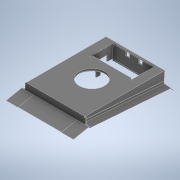
# Autodesk Inventor part: horni-cast
Saved by Autodesk Inventor 2022 (Build 260153000, 153)
## iProperties
Created: 2022-11-28
Part Number: horni-cast
Material: Generic
Document SubType Name: Modeling
Designer: matys
Density: 1 g/cm^3
Appearance: Gray
Author: matys
Autodesk Inventor part; units mm, degrees
ref_plane "YZ Plane" through (0, 0, 0) normal (1, 0, 0) x (0, 1, 0)
ref_plane "XZ Plane" through (0, 0, 0) normal (0, 1, 0) x (-1, 0, 0)
ref_plane "XY Plane" through (0, 0, 0) normal (0, 0, 1) x (1, 0, 0)
sketch "Sketch1" plane through (0, 0, 0) normal (0, 1, 0) x (-1, 0, 0)
  line L0 (0, 0) -> (0, -212.0143)
  line L1 (0, -212.0143) -> (140, -212.0143)
  line L2 (140, -212.0143) -> (140, 0)
  line L3 (140, 0) -> (0, 0)
  dimension "d0" = 212.0143
  dimension "d1" = 140
  constraints: 8 end point, 3 perpendicular, 1 vertical
  measures "d0" distance of L0.start L0.end
  measures "d1" distance of L0.end L1.end
extrude "Extrusion1" add sketch "Sketch1" along normal blind 2.5
sketch "Sketch2" plane through (0, 0, 0) normal (0, -1, 0) x (1, 0, 0)
  line L0 (0, 0) -> (0, -212.0143) projected
  line L1 (0, -212.0143) -> (0, -208.8143)
  line L2 (0, -212.0143) -> (-140, -212.0143) projected
  line L3 (-140, -208.8143) -> (-140, -212.0143)
  line L4 (-140, -212.0143) -> (0, -212.0143)
  line L5 (0, -212.0143) -> (0, -205.5643)
  line L6 (0, -205.5643) -> (-140, -205.5643)
  line L7 (-140, -205.5643) -> (-140, -212.0143)
  dimension "d5" = 6.45
  constraints: 12 end point, 3 perpendicular, 2 point on line
  measures "d5" distance of L0.end L5.end
extrude "Extrusion2" add sketch "Sketch2" along normal blind 40.4609
sketch "Sketch3" plane through (0, 2.5, 0) normal (1, 0, 0) x (0, 0, -1)
  line L0 (0, 0) -> (212.0143, 0) projected
  line L1 (212.0143, 0) -> (208.8143, 0)
  line L2 (212.0143, -42.9609) -> (205.5643, -42.9609) projected
  line L3 (208.8143, 0) -> (208.8143, -2.5)
  line L4 (205.5643, -2.5) -> (0, -2.5) projected
  line L5 (208.8143, -2.5) -> (205.5643, -2.5)
  line L6 (212.0143, 0) -> (209.3663, -37.8675)
  line L7 (212.0143, 0) -> (212.0143, -42.9609) projected
  line L8 (212.0143, 0) -> (209.3663, -37.8675)
  line L9 (209.3663, -37.8675) -> (205.5643, -37.8675)
  line L10 (205.5643, -2.5) -> (205.5643, -42.9609) projected
  line L11 (209.3663, -37.8675) -> (207.8663, -37.8675)
  line L12 (209.3663, -37.8675) -> (212.0143, -37.8675)
  line L13 (207.8663, -37.8675) -> (207.304, -40.3035)
  line L14 (207.304, -40.3035) -> (205.5643, -40.2123)
  line L15 (206.3702, -37.7629) -> (205.8078, -40.1988)
  line L16 (206.3702, -37.7629) -> (208.8143, -2.5)
  line L17 (212.0143, -42.9609) -> (205.5643, -42.9609)
  line L18 (205.5643, -42.9609) -> (205.5643, -2.5)
  line L19 (205.5643, -2.5) -> (212.0143, -2.5)
  line L20 (212.0143, -2.5) -> (212.0143, -42.9609)
  line L21 (212.0143, -2.5) -> (208.8143, -2.5)
  line L22 (208.8143, -2.5) -> (208.8143, 0)
  line L23 (208.8143, 0) -> (212.0143, 0)
  line L24 (212.0143, 0) -> (212.0143, -2.5)
  line L25 (205.8078, -40.1988) -> (205.7916, -40.2692)
  point P0 (206.3461, -37.8675)
  point P1 (205.8019, -40.2247)
  dimension "d8" = 3.2
  dimension "d9" = 86
  dimension "d10" = 37.8675
  dimension "d11" = 37.96
  dimension "d12" = 1.5
  dimension "d14" = 2.5
  dimension "d15" = 100
  dimension "d17" = 2.5
  constraints: 42 end point, 6 point on line, 4 parallel, 3 horizontal, 3 perpendicular, 1 vertical
  measures "d8" distance of L0.end L1.end
  measures "d9" angle of L0 L6
  measures "d10" vertical distance of L6.end L0.end
  measures "d11" distance of L6.end L0.end
  measures "d12" distance of L11.start L11.end
  measures "d14" distance of L13.start L13.end
  measures "d15" angle of L13 L14
  measures "d17" distance of L15.start L15.end
extrude "Extrusion3" cut sketch "Sketch3" against normal through all contours L7 L19 L6 | L16 L15 L9 L10 L5 | L19 L7 L12 L6 | L12 L7 L2 L10 L14 L13 L9 | L9 L15 L25 L14 L10
sketch "Sketch4" plane through (0, 2.5, -212.0143) normal (0, -0.0697565, -0.9975641) x (-1, 0, 0)
  line L0 (0, 0) -> (140, 0) projected
  line L1 (0, 0) -> (140, 0)
  line L2 (140, 0) -> (70, 0)
  line L3 (70, 0) -> (70, -46.5203)
  line L4 (70, 0) -> (120, 0)
  line L5 (120, 0) -> (120, -40.5339)
  line L6 (0, -40.5339) -> (140, -40.5339) projected
  line L7 (120, -40.5339) -> (20, -40.5339)
  line L8 (20, -40.5339) -> (20, 0)
  line L9 (0, -38.0646) -> (140, -38.0646) projected
  line L10 (20, -38.0646) -> (20, -33.0646)
  line L11 (0, -37.96) -> (0, 0) projected
  line L12 (0, -2.7171) -> (0, -38.0646) projected
  line L13 (0, -38.0646) -> (0, -30.0646)
  line L14 (0, -30.0646) -> (20, -30.0646)
  line L15 (0, -30.0646) -> (0, -29.0646)
  line L16 (0, -29.0646) -> (20, -29.0646)
  line L17 (0, -29.0646) -> (0, -46.3446)
  line L18 (0, -46.3446) -> (20, -46.3446)
  line L19 (20, -46.3446) -> (20, -40.5339)
  line L20 (0, -38.0646) -> (0, -40.5601) projected
  line L21 (0, -38.0646) -> (20, -37.96)
  point P0 (0, -17.2833)
  point P1 (0, -29.0646)
  point P2 (0, -38.0646)
  point P3 (0, -40.5339)
  point P4 (20, -40.5339)
  point P5 (0, -38.0646)
  dimension "d20" = 50
  dimension "d21" = 100
  dimension "d23" = 8
  dimension "d24" = 1
  dimension "d25" = 17.28
  constraints: 32 end point, 11 point on line, 6 perpendicular, 2 vertical, 1 collinear, 1 horizontal, 1 midpoint
  measures "d20" distance of L2.end L4.end
  measures "d21" distance of L5.end L7.end
  measures "d23" distance of L9.start L13.end
  measures "d24" distance of L13.end L15.end
  measures "d25" distance of L15.end L17.end
extrude "Extrusion4" add sketch "Sketch4" along normal blind 16 contours L8 L14 L11 L16 | L8 L21 L12 L11 L14 | L9 L21 L8 | L8 L6 L17 L9 | L19 L18 L17 L6
sketch "Sketch5" plane through (0, 2.5, 0) normal (1, 0, 0) x (0, 0, -1)
  line L0 (207.304, -40.3035) -> (207.8663, -37.8675) projected
  line L1 (207.8663, -37.8675) -> (209.3663, -37.8675) projected
  line L2 (207.8663, -37.8675) -> (209.3663, -37.8675)
  line L3 (209.9869, -28.9938) -> (225.9479, -30.1099) projected
  line L4 (209.3663, -37.8675) -> (209.9869, -28.9938)
  line L5 (209.9869, -28.9938) -> (209.9171, -29.9914)
  line L6 (212.0143, 0) -> (209.3663, -37.8675) projected
  line L7 (225.9479, -30.1099) -> (224.7425, -47.3478) projected
  line L8 (224.7425, -47.3478) -> (224.8122, -46.3503)
  line L9 (224.8122, -46.3503) -> (209.9869, -28.9938)
  line L10 (209.9869, -28.9938) -> (209.9171, -29.9914)
  line L11 (209.9171, -29.9914) -> (224.7425, -47.3478)
  line L12 (209.9869, -28.9938) -> (209.7776, -31.9865)
  line L13 (209.9869, -28.9938) -> (209.3663, -37.8675) projected
  line L14 (209.7776, -31.9865) -> (211.7384, -32.1236)
  line L15 (211.7384, -32.1236) -> (209.3663, -37.8675)
  line L16 (225.9479, -30.1099) -> (209.9869, -28.9938)
  line L17 (225.9479, -30.1099) -> (224.8122, -46.3503)
  line L18 (209.3663, -37.8675) -> (208.7815, -46.2317) projected
  line L19 (224.7425, -47.3478) -> (208.7815, -46.2317)
  line L20 (208.7815, -46.2317) -> (209.3663, -37.8675)
  point P0 (0, -2.5)
  dimension "d28" = 1
  dimension "d30" = 1
  dimension "d31" = 3
  constraints: 28 end point, 3 collinear, 3 perpendicular, 3 point on line, 1 horizontal
  measures "d28" distance of L3.start L5.end
  measures "d30" distance of L7.end L8.end
  measures "d31" distance of L3.start L12.end
extrude "Extrusion5" cut sketch "Sketch5" against normal through all contours L3 L7 L9 | L11 L19 L18 L15
sketch "Sketch7" plane through (0, 2.5, 0) normal (1, 0, 0) x (0, 0, -1)
  line L0 (209.9869, -28.9938) -> (209.3663, -37.8675) projected
  line L1 (209.9869, -28.9938) -> (209.3663, -37.8675)
  line L2 (209.3663, -37.8675) -> (211.7384, -32.1236)
  line L3 (224.7425, -47.3478) -> (211.7384, -32.1236) projected
  line L4 (211.7384, -32.1236) -> (224.7425, -47.3478)
  line L5 (209.9869, -28.9938) -> (224.8122, -46.3503) projected
  line L6 (224.7425, -47.3478) -> (224.8122, -46.3503)
  line L7 (224.8122, -46.3503) -> (209.9869, -28.9938)
  point P0 (0, -2.5)
  constraints: 10 end point, 3 collinear, 1 parallel
extrude "Extrusion6" add sketch "Sketch7" along normal blind 12
sketch "Sketch8" plane through (0, 0, 0) normal (0, -1, 0) x (1, 0, 0)
  line L0 (0, 0) -> (0, -2.5)
  line L1 (0, 0) -> (0, -208.8143) projected
  line L2 (0, -2.5) -> (-140, -2.5)
  line L3 (-140, -212.0143) -> (-140, 0) projected
  line L4 (-140, 0) -> (-140, -2.5)
  line L5 (0, 0) -> (0, 41.8054)
  line L6 (0, 41.8054) -> (-140, 41.8054)
  line L7 (-140, 0) -> (0, 0) projected
  line L8 (-140, 41.8054) -> (-140, 0)
  dimension "d37" = 2.5
  dimension "d38" = 41.8054
  constraints: 12 end point, 3 perpendicular, 2 point on line, 1 collinear, 1 vertical
  measures "d37" distance of L0.start L0.end
  measures "d38" distance of L0.start L5.end
extrude "Extrusion7" add sketch "Sketch8" along normal blind 27.8 and the other way blind 2.45
sketch "Sketch9" plane through (0, 2.5, 0) normal (1, 0, 0) x (0, 0, -1)
  line L0 (2.5, -30.3) -> (2.5, -2.5) projected
  line L1 (2.5, -2.5) -> (1.1835, -21.3273)
  line L2 (2.5, -2.5) -> (208.8143, -2.5) projected
  line L3 (2.5, -2.5) -> (1.3218, -19.3489)
  line L4 (0, 0) -> (212.0143, 0) projected
  line L5 (0, 0) -> (-1.2207, -17.4574)
  line L6 (-1.2207, -17.4574) -> (-41.8054, -25.3462)
  line L7 (-41.8054, -0.05) -> (-41.8054, -30.3) projected
  line L8 (-1.2207, -17.4574) -> (-38.1201, -24.6299)
  line L9 (1.1835, -21.3273) -> (-5.8352, -22.6916)
  line L10 (-5.8352, -22.6916) -> (-5.8352, -28.6916)
  line L11 (-41.8054, -0.05) -> (0, -0.05) projected
  line L12 (-41.8054, -0.05) -> (-41.8054, -25.4721)
  line L13 (-36.6554, -26.1524) -> (-41.6554, -26.1524)
  line L14 (-41.6554, -26.1524) -> (-41.8054, -25.3462)
  line L15 (-36.6554, -26.1524) -> (-36.5328, -28.4927)
  line L16 (-36.5328, -28.4927) -> (-35.0328, -28.4927)
  line L17 (-27.1023, -27.1504) -> (-5.8352, -28.6916)
  line L18 (-36.6554, -26.1524) -> (-27.1023, -27.1504)
  line L19 (-27.1023, -27.1504) -> (-35.0328, -28.4927)
  line L20 (-41.8054, -0.05) -> (2.5, -0.05)
  line L21 (2.5, -0.05) -> (2.5, -30.3)
  line L22 (2.5, -30.3) -> (-41.8054, -30.3)
  line L23 (-41.8054, -30.3) -> (-41.8054, -0.05)
  point P0 (0, -2.5)
  point P1 (-41.8054, -30.3)
  point P2 (-0.0035, -0.05)
  dimension "d43" = 94
  dimension "d44" = 16.89
  dimension "d45" = 17.5
  dimension "d46" = 94
  dimension "d47" = 105
  dimension "d49" = 7.15
  dimension "d50" = 105
  dimension "d51" = 6
  dimension "d52" = 25.4221
  dimension "d56" = 5
  dimension "d57" = 2.3435
  dimension "d58" = 93
  dimension "d59" = 1.5
  dimension "d60" = 9.6051
  constraints: 38 end point, 4 point on line, 2 horizontal, 2 parallel, 1 perpendicular, 1 vertical
  measures "d43" angle of L2 L1
  measures "d44" distance of L0.end L3.end
  measures "d45" distance of L4.start L5.end
  measures "d46" angle of L4 L5
  measures "d47" angle of L6 L5
  measures "d49" distance of L1.end L9.end
  measures "d50" angle of L1 L9
  measures "d51" distance of L9.end L10.end
  measures "d52" distance of L7.start L12.end
  measures "d56" distance of L13.start L13.end
  measures "d57" distance of L13.start L15.end
  measures "d58" angle of L13 L15
  measures "d59" distance of L15.end L16.end
  measures "d60" distance of L17.start L13.start
extrude "Extrusion8" cut sketch "Sketch9" against normal through all contours L22 L7 L14 L13 L15 L16 L19 L17 L10 L9 L1 L0 | L7 L11 L5 L6
sketch "Sketch11" plane through (0, 2.5, 0) normal (0, 1, 0) x (1, 0, 0)
  line L0 (-140, -41.8054) -> (-140, -1.2207) projected
  line L1 (0, -1.2207) -> (-140, -1.2207) projected
  line L2 (-140, -1.2207) -> (0, -1.2207)
  line L3 (0, -1.2207) -> (-70, -1.2207)
  line L4 (-70, -1.2207) -> (-20, -1.2207)
  line L5 (-20, -1.2207) -> (-120, -1.2207)
  line L6 (0, -41.6554) -> (-140, -41.6554) projected
  line L7 (-120, -1.2207) -> (-20, -1.2207)
  line L8 (-20, -1.2207) -> (-20, -41.6554)
  line L9 (-20, -41.6554) -> (-120, -41.6554)
  line L10 (-120, -41.6554) -> (-120, -1.2207)
  line L11 (-140, -1.2207) -> (0, -1.2207)
  line L12 (0, -1.2207) -> (0, -41.6554)
  line L13 (0, -41.6554) -> (-140, -41.6554)
  line L14 (-140, -41.6554) -> (-140, -1.2207)
  line L15 (-140, -1.2207) -> (0, -1.2207)
  line L16 (0, -1.2207) -> (0, -57.5957)
  line L17 (0, -57.5957) -> (-140, -57.5957)
  line L18 (-140, -57.5957) -> (-140, -1.2207)
  line L19 (-120, -41.6554) -> (-120, -57.5957)
  line L20 (-20, -41.6554) -> (-20, -57.5957)
  point P0 (0, 0)
  point P1 (0, -1.2207)
  point P2 (0, -41.6554)
  dimension "d65" = 50
  dimension "d66" = 100
  constraints: 36 end point, 8 equal length, 5 point on line, 4 perpendicular, 3 horizontal, 1 midpoint
  measures "d65" distance of L3.end L4.end
  measures "d66" distance of L4.end L5.end
extrude "Extrusion9" cut sketch "Sketch11" against normal through all contours L0 L6 L19 L17 L18 | L0 L1 L10 L6 | L8 L1 L12 L6 | L6 L16 L17 L20
sketch "Sketch12" plane through (-20, -26.1916, 5.8352) normal (1, 0, 0) x (0, 0, -1)
  line L0 (-35.9702, 3.3454) -> (4.6144, 11.2342) projected
  line L1 (4.6144, 11.2342) -> (4.6144, 11.0342)
  line L2 (4.6144, 6.897) -> (4.6144, 11.2342) projected
  line L3 (-35.9702, 3.3454) -> (-35.8788, 2.8538)
  line L4 (-35.9702, 3.3454) -> (-35.8202, 2.5392) projected
  line L5 (-35.8788, 2.8538) -> (4.6144, 11.0342)
  line L6 (-35.8788, 2.8538) -> (-34.3594, 3.1608)
  line L7 (-34.3594, 3.1608) -> (-36.8589, 2.6558)
  line L8 (-36.8589, 2.6558) -> (-36.3688, 2.7548)
  line L9 (-36.3688, 2.7548) -> (-36.3688, 2.2548)
  line L10 (4.6144, 11.0342) -> (4.6144, 10.2342)
  line L11 (4.6144, 10.2342) -> (-36.3688, 2.2548)
  line L12 (4.6144, 10.2342) -> (-4.5716, 8.4457)
  line L13 (4.6144, 10.2342) -> (6.0868, 10.5209)
  line L14 (6.0868, 10.5209) -> (6.0868, 11.3209)
  line L15 (4.6144, 11.2342) -> (4.6144, 6.897) projected
  line L16 (6.0868, 11.3209) -> (4.6144, 11.0342)
  point P0 (5.8352, 26.1916)
  dimension "d69" = 0.2
  dimension "d70" = 0.5
  dimension "d71" = 2.55
  dimension "d72" = 0.5
  dimension "d73" = 0.5
  dimension "d74" = 0.8
  dimension "d97" = 1.5
  dimension "d98" = 0.8
  constraints: 26 end point, 8 point on line, 1 parallel, 1 vertical
  measures "d69" distance of L0.end L1.end
  measures "d70" distance of L0.start L3.end
  measures "d71" distance of L6.end L7.end
  measures "d72" distance of L7.end L8.end
  measures "d73" distance of L8.end L9.end
  measures "d74" distance of L1.end L10.end
  measures "d97" distance of L10.end L13.end
  measures "d98" distance of L13.end L14.end
extrude "Extrusion10" add sketch "Sketch12" along normal blind 32 contours L5 L2 L11 L9 L7 | L16 L14 L13 L2
sketch "Sketch13" plane through (0, 2.5, 0) normal (1, 0, 0) x (0, 0, -1)
  line L0 (207.8663, -37.8675) -> (209.3663, -37.8675) projected
  line L1 (209.9869, -28.9938) -> (212.0143, 0) projected
  line L2 (209.3663, -37.8675) -> (209.9869, -28.9938)
  line L3 (-1.2207, -17.4574) -> (-1.2207, -21.7947) projected
  line L4 (-1.2207, -21.7947) -> (209.3663, -37.8675)
  line L5 (209.9869, -28.9938) -> (209.3663, -37.8675) projected
  line L6 (209.9869, -28.9938) -> (-0.9019, -12.8979)
  line L7 (-1.2207, -17.4574) -> (-1.2207, -21.7947)
  line L8 (-1.2207, -17.4574) -> (-0.0035, -0.05) projected
  line L9 (-0.9019, -12.8979) -> (-1.2207, -17.4574)
  line L10 (-0.9019, -12.8979) -> (1.7587, -13.101)
  line L11 (2.5, -2.5) -> (1.1835, -21.3273) projected
  line L12 (-1.2207, -17.4574) -> (1.4262, -17.4574)
  line L13 (1.4262, -17.4574) -> (0.1027, -17.4574)
  line L14 (0.4284, -12.9995) -> (0.4284, -17.4574)
  line L15 (0.4284, -17.4574) -> (0.4284, -21.9205)
  line L16 (209.9869, -28.9938) -> (209.3663, -37.8675)
  point P0 (0, -2.5)
  point P1 (-1.2207, -18.4574)
  constraints: 22 end point, 7 point on line, 2 collinear, 2 midpoint, 1 horizontal, 1 parallel, 1 perpendicular, 1 vertical
extrude "Extrusion11" add sketch "Sketch13" along normal blind 12 contours L4 L15 L14 L6 L2
sketch "Sketch14" plane through (0, 2.5, 0) normal (1, 0, 0) x (0, 0, -1)
  line L0 (-41.7139, -25.8378) -> (-1.2207, -17.6574) projected
  line L1 (-1.2207, -17.4574) -> (-1.2207, -17.6574) projected
  line L2 (-1.2207, -17.6574) -> (-1.2207, -17.4574)
  line L3 (212.0143, 0) -> (0, 0) projected
  line L4 (-1.2207, -17.4574) -> (0, 0)
  line L5 (-1.2207, -17.6574) -> (-1.2207, -18.4574) projected
  line L6 (-1.2207, -18.4574) -> (-1.2207, -21.7947) projected
  line L7 (-1.2207, -17.6574) -> (-1.2207, -21.7947)
  line L8 (-1.2207, -21.7947) -> (0.4284, -21.4741) projected
  line L9 (-1.2207, -21.7947) -> (0.4284, -21.4741)
  line L10 (0.4284, -12.9995) -> (0.4284, -21.9205) projected
  line L11 (0.4284, -21.4741) -> (0.4284, -12.9995)
  line L12 (0.4284, -12.9995) -> (1.3309, -0.0931)
  line L13 (1.3309, -0.0931) -> (1.3374, 0)
  line L14 (0, -0.05) -> (0, 0) projected
  line L15 (0, 0) -> (1.3374, 0)
  line L16 (-0.0035, -0.05) -> (-1.2207, -17.4574) projected
  line L17 (0, 0) -> (-1.2207, -17.4574)
  point P0 (0, -2.5)
  constraints: 18 end point, 4 collinear, 2 point on line, 1 vertical
extrude "Extrusion12" add sketch "Sketch14" along normal blind 3
fillet "Fillet1" radius 1.5 1 edges at (3, 2.5, -0.6687)
chamfer "Chamfer1" distance 8.5 distance2 11 1 edges at (12, -18.4967, -105.2076) measured on face at (12, -18.9952, -105.1696)
sketch "Sketch17" plane through (12, 2.5, 0) normal (1, 0, 0) x (0, 0, -1)
  line L0 (211.7384, -32.1236) -> (209.3663, -37.8675) projected
  line L1 (216.7901, -38.0378) -> (217.7763, -38.1131) projected
  line L2 (209.525, -37.4833) -> (216.7901, -38.0378)
  line L3 (211.7384, -32.1236) -> (216.7901, -38.0378) projected
  line L4 (216.7901, -38.0378) -> (211.7384, -32.1236)
  line L5 (211.7384, -32.1236) -> (209.525, -37.4833)
  point P0 (0, -2.5)
  constraints: 6 end point, 2 collinear, 1 point on line
extrude "Extrusion14" add sketch "Sketch17" against normal blind 12
sketch "Sketch20" plane through (4.8661, -29.6236, -211.7384) normal (0, 0.381702, 0.9242854) x (1, 0, 0)
  line L0 (7.1339, -3.2313) -> (-3.8661, 2.2243) projected
  line L1 (-3.8661, 2.2243) -> (7.1339, -3.2313)
  line L2 (7.1339, 0) -> (7.1339, -5.7987) projected
  line L3 (7.1339, -3.2313) -> (7.1339, 0)
  line L4 (7.1339, 0) -> (0.6187, 0)
  point P0 (-4.8661, -53.4403)
  point P1 (0.6187, 0)
  constraints: 6 end point, 2 collinear, 1 perpendicular, 1 point on line
extrude "Extrusion15" cut sketch "Sketch20" against normal through all
sketch "Sketch23" plane through (0, -19.4205, -0.4284) normal (0, 0, 1) x (1, 0, 0)
  point P0 (0, 19.4205)
sketch "Sketch24" plane through (1, -10.4995, -0.4284) normal (0.6114475, 0.7889903, -0.060219) x (0.791285, -0.6096743, 0.0465328)
  line L0 (13.9014, 210.3535) -> (4.8858, 212.1526) projected
  line L1 (4.8858, 212.1526) -> (13.9014, 217.6398) projected
  line L2 (4.8858, 212.1526) -> (13.9014, 217.6398)
  line L3 (13.9014, 210.3535) -> (13.9014, 217.6398) projected
  line L4 (13.9014, 217.6398) -> (13.9014, 210.3535)
  line L5 (13.9014, 210.3535) -> (4.8858, 212.1526)
  point P0 (-7.1726, -1.2262)
  constraints: 6 end point, 2 collinear
extrude "Extrusion16" cut sketch "Sketch24" along normal blind 10
chamfer "Chamfer2" distance 0.395 distance2 11 1 edges at (12, -27.394, -104.8974) measured on face at (12, -27.2943, -104.905)
sketch "Sketch26" plane through (0, -10.601, -1.7587) normal (0, 0.9971, -0.0761027) x (1, 0, 0)
  line L0 (12, 217.2946) -> (1, 208.8338) projected
  line L1 (1, 208.8338) -> (0, 208.8338)
  line L2 (0, -0.6553) -> (0, 205.8941) projected
  line L3 (0, 208.8338) -> (0, -0.6553)
  line L4 (1, -0.6553) -> (1, 208.8904) projected
  line L5 (0, -0.6553) -> (1, -0.6553)
  line L6 (1, -0.6553) -> (1, 208.8338)
  line L7 (0, -1.3342) -> (0, 0) projected
  line L8 (0, -0.6553) -> (0, -1.3342)
  line L9 (0, -1.3342) -> (1, -1.3342) projected
  line L10 (0, -1.3342) -> (1, -1.3342)
  line L11 (1, -1.3342) -> (1, -0.6553)
  point P0 (0, -2.5604)
  point P1 (0, 205.8941)
  constraints: 14 end point, 4 perpendicular, 2 collinear, 1 horizontal
extrude "Extrusion17" add sketch "Sketch26" along normal blind 6
sketch "Sketch27" plane through (0, 0, -2.5) normal (1, 0, 0) x (0, 0, -1)
  line L0 (-1.1626, 2.5) -> (-1.2675, 1) projected
  line L1 (-1.615, -4.5169) -> (207.9435, -20.5112) projected
  line L2 (-1.1626, 2.5) -> (-1.615, -4.5169)
  line L3 (-1.615, -4.5169) -> (207.9435, -20.5112)
  line L4 (209.5143, 2.5) -> (-2.5, 2.5) projected
  line L5 (207.9435, -20.5112) -> (209.5143, 2.5)
  line L6 (209.5143, 2.5) -> (-1.1626, 2.5)
  line L7 (206.3143, 0) -> (0, 0) projected
  point P0 (-2.5, 0)
  constraints: 8 end point, 1 collinear, 1 parallel
extrude "Extrusion18" add sketch "Sketch27" along normal blind 0.5 and the other way blind 2.5
sketch "Sketch29" plane through (-20, -26.1916, 5.8352) normal (1, 0, 0) x (0, 0, -1)
  line L0 (-36.3688, 2.2548) -> (-34.9083, 2.5392) projected
  line L1 (6.0868, 10.5209) -> (6.0868, 11.3209) projected
  line L2 (-36.3688, 2.2548) -> (6.0868, 10.5209)
  line L3 (6.0868, 10.5209) -> (6.2636, 10.5209)
  line L4 (6.2636, 14.1422) -> (6.2636, 7.2175) projected
  line L5 (4.6144, 10.2342) -> (4.6144, 6.897) projected
  line L6 (4.6144, 10.2342) -> (4.6144, 6.897)
  line L7 (0, 6) -> (4.6144, 6.897) projected
  line L8 (4.6144, 6.897) -> (0, 6)
  line L9 (0, 6) -> (0, -4.6207)
  line L10 (0, -4.6207) -> (-37.0061, -4.3774)
  line L11 (-37.0061, -4.3774) -> (-36.3688, 2.2548)
  line L12 (-36.3688, 2.2548) -> (6.0868, 10.5209) projected
  line L13 (4.6144, 10.2342) -> (6.0868, 10.5209)
  line L14 (6.0868, 10.5209) -> (6.2636, 10.5209)
  line L15 (6.2636, 7.2175) -> (7.0186, 7.3643) projected
  line L16 (6.2636, 7.2175) -> (4.6144, 6.897)
  line L17 (4.6144, 11.2342) -> (4.6144, 6.897) projected
  line L18 (4.6144, 10.2342) -> (4.6144, 6.897)
  point P0 (5.8352, 26.1916)
  constraints: 22 end point, 4 collinear, 1 horizontal, 1 parallel, 1 perpendicular, 1 point on line, 1 vertical
extrude "Extrusion19" cut sketch "Sketch29" along normal blind 40 and the other way blind 2
sketch "Sketch30" plane through (0, -35.3675, -207.8663) normal (1, 0, 0) x (0, 0, -1)
  line L0 (-0.5624, -2.4359) -> (0, 0)
  line L1 (0, 0) -> (1.5, 0) projected
  line L2 (0, 0) -> (1.5, 0)
  line L3 (1.5, 0) -> (1.725, 0.9744)
  line L4 (1.725, 0.9744) -> (-1.4358, 0.9744)
  line L5 (-0.4576, 15.0879) -> (-1.4876, 0.228) projected
  line L6 (-2.0645, -2.3572) -> (-0.5624, -2.4359) projected
  line L7 (-0.5624, -2.4359) -> (-2.0645, -2.3572)
  line L8 (-1.4876, 0.228) -> (-1.4961, 0.1046) projected
  line L9 (-2.0645, -2.3572) -> (-1.4961, 0.1046)
  line L10 (-1.4961, 0.1046) -> (-1.4391, 1.1917)
  line L11 (3.8721, 5.7439) -> (1.6587, 0.3842) projected
  line L12 (-1.4391, 1.1917) -> (1.6587, 0.3842)
  point P0 (-207.8663, 35.3675)
  point P1 (1.5927, 0.4014)
  point P2 (-0.6054, 0.9744)
  dimension "d109" = 1
  constraints: 16 end point, 3 parallel, 2 collinear, 1 perpendicular, 1 point on line
  measures "d109" distance of L1.end L3.end
extrude "Extrusion20" cut sketch "Sketch30" against normal blind 22.2 contours L6 L9 L8 L5 L4 L12 L3 L1 L0
sketch "Sketch31" plane through (-22, -26.1916, 5.8352) normal (1, 0, 0) x (0, 0, -1)
  line L0 (7.0186, 7.3643) -> (4.6144, 6.897) projected
  line L1 (6.2642, 7.2176) -> (0, 7.2176)
  line L2 (0, 6) -> (4.6144, 6.897) projected
  line L3 (0, 6) -> (0, 7.2176)
  point P0 (5.8352, 26.1916)
  constraints: 4 end point, 1 horizontal, 1 perpendicular, 1 point on line
extrude "Extrusion21" cut sketch "Sketch31" against normal through all
sketch "Sketch32" plane through (-22, -18.974, -0.4284) normal (0, -1, 0) x (1, 0, 0)
  point P0 (22, 0.4284)
sketch "Sketch33" plane through (-22, -26.1916, 5.8352) normal (1, 0, 0) x (0, 0, -1)
  line L0 (6.0868, 10.5209) -> (6.0868, 11.3209) projected
  line L1 (6.0868, 10.5209) -> (-32.0303, 10.5209)
  line L2 (-29.1976, 0.1989) -> (-21.2671, 1.5413) projected
  line L3 (-29.1976, 0.1989) -> (-29.1976, 10.5209)
  line L4 (4.6144, 7.2176) -> (0, 7.2176) projected
  line L5 (0, 7.2176) -> (86.25, 7.2176)
  line L6 (86.25, 7.2176) -> (86.25, 26.1916)
  line L7 (214.6495, 26.1916) -> (8.3352, 26.1916) projected
  line L8 (8.3352, 26.1916) -> (8.0124, 21.5761) projected
  line L9 (86.25, 26.1916) -> (8.3352, 26.1916)
  line L10 (8.3352, 26.1916) -> (7.0084, 7.2176)
  line L11 (6.2636, 10.5209) -> (6.2636, 7.2176) projected
  line L12 (6.0868, 10.5209) -> (6.2636, 10.5209) projected
  line L13 (6.2636, 10.5209) -> (6.0868, 10.5209)
  line L14 (6.0868, 10.5209) -> (0, 9.3358)
  line L15 (-34.9083, 2.5392) -> (6.0868, 10.5209) projected
  line L16 (0, 7.2176) -> (0, 0) projected
  line L17 (0, 9.3358) -> (0, 7.2176)
  line L18 (0, 7.2176) -> (6.2636, 7.2176) projected
  line L19 (0, 7.2176) -> (6.2636, 7.2176)
  line L20 (6.2636, 7.2176) -> (6.2636, 10.5209)
  line L21 (-35.8202, 2.5392) -> (-30.8202, 2.5392) projected
  line L22 (-30.8202, 2.5392) -> (0, 2.5392)
  line L23 (0, 2.5392) -> (0, 7.2176)
  line L24 (0, 9.3358) -> (-27.8909, 3.9055)
  line L25 (-30.8202, 2.5392) -> (-34.9083, 2.5392) projected
  line L26 (-34.9083, 2.5392) -> (-30.8202, 2.5392)
  line L27 (-30.8202, 2.5392) -> (-34.9083, 2.5392)
  line L28 (-27.8909, 3.9055) -> (-34.9083, 2.5392)
  line L29 (215.2015, -9.1759) -> (213.7015, -9.1759) projected
  line L30 (-30.8202, 2.5392) -> (215.2015, -9.1759)
  line L31 (0, 2.5392) -> (0, 1.0716)
  line L32 (6.2636, 6.7711) -> (215.2015, -9.1759) projected
  line L33 (215.2015, -9.1759) -> (198.7809, -8.394)
  line L34 (198.7809, -8.394) -> (198.7809, 26.1916)
  line L35 (214.6495, 26.1916) -> (8.3352, 26.1916) projected
  line L36 (215.2307, -8.7579) -> (215.2015, -9.1759) projected
  line L37 (215.2015, -9.1759) -> (215.2307, -8.7579)
  line L38 (215.2307, -8.7579) -> (215.2161, -8.9669)
  line L39 (215.2161, -8.9669) -> (198.7809, 1010.7633)
  line L40 (198.7809, 26.1916) -> (214.6495, 26.1916)
  line L41 (212.2054, -9.0713) -> (212.2657, -8.2015) projected
  line L42 (214.6495, 26.1916) -> (212.9734, -9.0059)
  line L43 (6.2636, 6.7711) -> (215.2015, -9.1759) projected
  line L44 (212.9704, -9.0697) -> (212.9734, -9.0059)
  line L45 (215.2015, -9.1759) -> (215.2307, -8.7579)
  line L46 (215.2307, -8.7579) -> (215.2161, -8.9669)
  line L47 (198.7809, -8.394) -> (198.7809, -8.194)
  line L48 (215.2161, -8.9669) -> (198.7809, -8.194)
  line L49 (86.25, 7.2176) -> (198.7809, 7.2176)
  line L50 (86.25, 26.1916) -> (198.7809, 26.1916)
  point P0 (5.8352, 26.1916)
  point P1 (-29.1976, 2.4619)
  point P2 (-29.1976, 2.5392)
  point P3 (198.7809, -7.9226)
  point P4 (215.2161, -8.9669)
  point P5 (198.7809, -8.1843)
  dimension "d114" = 86.25
  dimension "d117" = 16.4392
  dimension "d118" = 0.2
  constraints: 66 end point, 19 point on line, 11 collinear, 6 perpendicular, 3 vertical, 2 horizontal, 1 midpoint, 4 other
  measures "d114" distance of L4.end L5.end
  measures "d117" distance of L29.start L33.end
  measures "d118" distance of L33.end L47.end
extrude "Extrusion22" add sketch "Sketch33" along normal blind 2 contours L12 L11 L5 L4 L17 L14 | L17 L16 L22 L3 L15 | L3 L22 L21 L15 | L22 L16 L30 L3 | L10 L8 L7 L6 L5 | L6 L7 L34 L49 | L34 L7 L42 L48 L32 | L32 L48 L34 | L39 L48 L42
sketch "Sketch34" plane through (0, 2.5, 0) normal (0, 1, 0) x (1, 0, 0)
  line L0 (-2.5, 212.0143) -> (-140, 212.0143) projected
  line L1 (-140, 212.0143) -> (-140, 129.7851)
  line L2 (-140, 208.8143) -> (-140, 2.5) projected
  line L3 (-140, 129.7851) -> (-2.5, 129.7851)
  line L4 (-2.5, 207.4087) -> (-2.5, 2.1773) projected
  line L5 (-2.5, 129.7851) -> (0, 129.7851)
  line L6 (0.5, 212.0143) -> (0.5, 1.3374) projected
  line L7 (0.5, 129.7851) -> (0, 129.7851)
  line L8 (-20, -41.6554) -> (-120, -41.6554) projected
  line L9 (-120, -41.6554) -> (-20, -41.6554)
  line L10 (-20, -41.6554) -> (-70, -41.6554)
  line L11 (-70, -41.6554) -> (-70, 212.0143)
  line L12 (-70, 80.2843) -> (-140, 80.2843)
  line L13 (-140, 80.2843) -> (1, 80.2843)
  line L14 (1, 0.885) -> (1, 210.4435) projected
  line L15 (-70, 80.2843) -> (-70, 105.0347)
  line L16 (-70, 105.0347) -> (-70, 91.5347)
  line L17 (-70, 91.5347) -> (-70, 50.5347)
  line L18 (-70, 129.7851) -> (-70, 62.7851)
  line L19 (-70, 129.7851) -> (-70, 96.2851)
  circle A0 centre (-70, 96.2851) radius 33.5
  point P0 (0, 0)
  dimension "d119" = 82.2292
  dimension "d125" = 67
  constraints: 28 end point, 14 point on line, 4 perpendicular, 2 coincident, 2 midpoint, 1 collinear, 1 horizontal, 1 vertical alignment, 2 other
  measures "d119" distance of L0.end L1.end
  measures "d125" distance of L18.start L18.end
extrude "Extrusion23" cut sketch "Sketch34" against normal blind 5 contours A0 L13 L11 | L11 L12 A0 | L12 L11 A0 | A0 L11 L13
sketch "Sketch35" plane through (0, 0, 0) normal (0, -1, 0) x (1, 0, 0)
  circle A0 centre (-70, -96.2851) radius 33.5 projected
  circle A1 centre (-70, -96.2851) radius 33.5
  line L0 (-36.5, -96.2851) -> (-28.5, -96.2851)
  circle A2 centre (-70, -96.2851) radius 41.5
  point P0 (0, 0)
  dimension "d126" = 8
  constraints: 2 coincident, 2 end point, 2 horizontal alignment, 1 horizontal, 4 other
  measures "d126" distance of L0.start L0.end
extrude "Extrusion24" add sketch "Sketch35" along normal blind 2.5
sketch "Sketch36" plane through (-70, -2.5, -96.2851) normal (0, -1, 0) x (1, 0, 0)
  circle A0 centre (0, 0) radius 33.5 projected
  line L0 (33.5, 0) -> (38.5, 0)
  circle A1 centre (0, 0) radius 38.5
  circle A2 centre (0, 0) radius 41.5
  point P0 (70, 96.2851)
  dimension "d129" = 5
  constraints: 2 coincident, 2 end point, 2 horizontal alignment, 1 centre point, 1 horizontal, 3 other
  measures "d129" distance of L0.start L0.end
extrude "Extrusion25" add sketch "Sketch36" along normal blind 5 contours A2
sketch "Sketch37" plane through (-70, -7.5, -96.2851) normal (0, -1, 0) x (1, 0, 0)
  circle A0 centre (0, 0) radius 41.5 projected
  line L0 (0, 41.5) -> (0, 30)
  circle A1 centre (0, 0) radius 30
  circle A2 centre (0, 0) radius 41.5
  point P0 (70, 96.2851)
  dimension "d132" = 11.5
  constraints: 3 vertical alignment, 2 coincident, 2 end point, 1 vertical, 5 other
  measures "d132" distance of L0.start L0.end
extrude "Extrusion26" add sketch "Sketch37" along normal blind 3
sketch "Sketch38" plane through (0, 0, 0) normal (0, -1, 0) x (1, 0, 0)
  circle A0 centre (-70, -96.2851) radius 41.5 projected
  circle A1 centre (-70, -96.2851) radius 41.5
  line L0 (-28.5, -96.2851) -> (-18, -96.2851)
  line L1 (-70, -44.2851) -> (-22, -44.2851)
  line L2 (-70, -148.2851) -> (-22, -148.2851)
  line L3 (-22, -148.2851) -> (-22, -96.2851)
  line L4 (-22, -44.2851) -> (-22, -96.2851)
  line L5 (-70, -44.2851) -> (-70, -148.2851)
  line L6 (-70, -44.2851) -> (-118, -44.2851)
  line L7 (-70, -148.2851) -> (-118, -148.2851)
  line L8 (-118, -148.2851) -> (-118, -96.2851)
  line L9 (-118, -44.2851) -> (-118, -96.2851)
  arc A2 (-22, -76.2851) -> (-118, -76.2851) centre (-70, -96.2851) ccw
  arc A3 (-118, -116.2851) -> (-22, -116.2851) centre (-70, -96.2851) ccw
  point P0 (0, 0)
  dimension "d135" = 10.5
  constraints: 20 end point, 6 point on circle, 5 point on line, 3 symmetric about line, 2 centre point, 2 coincident, 2 horizontal, 1 horizontal alignment, 1 parallel, 1 perpendicular, 1 tangent, 1 vertical, 2 other
  measures "d135" distance of L0.start L0.end
extrude "Extrusion27" add sketch "Sketch38" along normal blind 10.5 contours L0 L3 A3 L5 A0 | A0 L5 A2 L4 L0 | A0 L5 A3 L8 L9 A2 | A2 L9 L6 | L1 L4 A2 | A3 L3 L2 | L7 L8 A3
chamfer "Chamfer3" distance 10.5 distance2 10.5 1 edges at (-70, -10.5, -44.2851) measured on face at (-70, -10.5, -44.7851)
chamfer "Chamfer4" distance 10.5 distance2 10.5 1 edges at (-70, -10.5, -148.2851) measured on face at (-70, -10.5, -147.7851)
sketch "Sketch39" plane through (0, 2.5, 0) normal (0, 1, 0) x (1, 0, 0)
  circle A0 centre (-70, 96.2851) radius 30 projected
  line L0 (-70, 96.2851) -> (-70, 263.3995)
  line L1 (-70, 263.3995) -> (-156.8416, 263.3995)
  line L2 (-156.8416, 263.3995) -> (-156.8416, -86.9527)
  line L3 (-156.8416, -86.9527) -> (-70, -86.9527)
  line L4 (-70, -86.9527) -> (-70, 263.3995)
  point P0 (0, 0)
  point P1 (-70, 66.2851)
  point P2 (-70, 126.2851)
  constraints: 10 end point, 2 parallel, 1 horizontal, 1 perpendicular, 1 vertical
extrude "Extrusion28" cut sketch "Sketch39" against normal through all contours A0 L4 L3 L2 L1 L0
mirror "Mirror1" about plane through (-70, 2.5, -263.3995) normal (-1, 0, 0)
sketch "Sketch40" plane through (0, 2.5, 0) normal (0, 1, 0) x (1, 0, 0)
  line L0 (-140.5, 210.4435) -> (-140.5, 212.0143) projected
  line L1 (-140.5, 212.0143) -> (-136.5, 212.0143)
  line L2 (-140.5, 212.0143) -> (-137.5, 212.0143) projected
  line L3 (-136.5, 212.0143) -> (-136.5, 207.0143)
  line L4 (-120, 206.4305) -> (-140, 206.4305) projected
  line L5 (-136.5, 207.0143) -> (0, 207.0143)
  line L6 (0, 0.4284) -> (0, 209.3663) projected
  line L7 (0, 207.0143) -> (-4, 207.0143)
  line L8 (-4, 207.0143) -> (-4, 150.2143)
  line L9 (-4, 150.2143) -> (-136.5, 150.2143)
  line L10 (-136.5, 150.2143) -> (-136.5, 207.0143)
  line L11 (-136.5, 150.2143) -> (-118, 150.2143)
  line L12 (-118, 1.1732) -> (-118, 192.9458) projected
  line L13 (-4, 150.2143) -> (-22.5, 150.2143)
  line L14 (-22.5, 150.2143) -> (-22.5, 207.0143)
  line L15 (-117.8, 206.4305) -> (-118, 206.4305) projected
  line L16 (-22.5, 207.0143) -> (-21, 207.0143)
  line L17 (-21, 207.0143) -> (-21, 150.2143)
  line L18 (-118, 150.2143) -> (-119.5, 150.2143)
  line L19 (-119.5, 150.2143) -> (-119.5, 207.0143)
  line L20 (-118, 208.8143) -> (-118, 148.2851) projected
  line L21 (-118, 150.2143) -> (-118, 208.8143)
  line L22 (-4, 207.0143) -> (-22, 207.0143)
  line L23 (-22, 208.8143) -> (-22, 148.2851) projected
  line L24 (-22, 1.1732) -> (-22, 192.9458) projected
  line L25 (-22, 207.0143) -> (-22.5, 150.2143)
  line L26 (-136.5, 207.0143) -> (-101.5, 207.0143)
  line L27 (-101.5, 207.0143) -> (-101.5, 150.2143)
  line L28 (-4, 207.0143) -> (-39, 207.0143)
  line L29 (-39, 207.0143) -> (-39, 150.2143)
  point P0 (0, 0)
  point P1 (-118.2052, 207.0143)
  point P2 (-118, 207.0143)
  dimension "d146" = 4
  dimension "d147" = 5
  dimension "d148" = 4
  dimension "d149" = 56.8
  dimension "d150" = 18.5
  dimension "d151" = 1.5
  dimension "d152" = 1.5
  dimension "d155" = 35
  dimension "d156" = 35
  constraints: 40 end point, 10 point on line, 6 perpendicular, 4 vertical, 2 collinear, 10 other
  measures "d146" distance of L0.end L1.end
  measures "d147" distance of L1.end L3.end
  measures "d148" distance of L7.start L7.end
  measures "d149" distance of L7.end L8.end
  measures "d150" distance of L8.end L13.end
  measures "d151" distance of L14.end L16.end
  measures "d152" distance of L11.end L18.end
  measures "d155" distance of L3.end L26.end
  measures "d156" distance of L7.end L28.end
extrude "Extrusion29" cut sketch "Sketch40" against normal blind 10 contours L5 L27 L9 L12 L20 | L5 L29 L9 L27 | L5 L14 L9 L29 | L5 L25 L14
sketch "Sketch41" plane through (0, 2.5, 0) normal (0, 1, 0) x (1, 0, 0)
  circle A0 centre (-70, 96.2851) radius 33.5 projected
  line L0 (-70, 96.2851) -> (-70, 257.496)
  line L1 (-70, 257.496) -> (-179.0373, 257.496)
  line L2 (-179.0373, 257.496) -> (-179.0373, -116.1167)
  line L3 (-179.0373, -116.1167) -> (-70, -116.1167)
  line L4 (-70, -116.1167) -> (-70, 96.2851)
  point P0 (0, 0)
  point P1 (-70, 62.7851)
  point P2 (-70, 129.7851)
  constraints: 10 end point, 3 perpendicular, 1 collinear, 1 point on line, 1 vertical
extrude "Extrusion30" cut sketch "Sketch41" against normal through all contours L0 L4 A0 | A0 L4 L3 L2 L1 L0 picked at (-72.6724, 74.2762)
sketch "Sketch42" plane through (-70, 2.5, -62.7851) normal (-1, 0, 0) x (0, 0, 1)
  line L0 (104.5905, -25.3462) -> (64.0058, -17.4574) projected
  line L1 (104.4405, -26.1524) -> (104.499, -25.8378) projected
  line L2 (104.5905, -25.3462) -> (104.4405, -26.1524)
  line L3 (99.3179, -28.4927) -> (99.4405, -26.1524) projected
  line L4 (104.4405, -26.1524) -> (99.4405, -26.1524)
  line L5 (99.4405, -26.1524) -> (99.3179, -28.4927)
  line L6 (99.3179, -28.4927) -> (97.8179, -28.4927)
  line L7 (89.8874, -27.1504) -> (97.8179, -28.4927) projected
  line L8 (97.8179, -28.4927) -> (89.8874, -27.1504)
  line L9 (89.8874, -27.1504) -> (68.6203, -28.6916) projected
  line L10 (89.8874, -27.1504) -> (68.6203, -28.6916)
  line L11 (68.6203, -21.474) -> (62.3567, -21.474) projected
  line L12 (68.6203, -28.6916) -> (68.6203, -21.474)
  line L13 (68.6203, -21.474) -> (62.3561, -21.474) projected
  line L14 (68.6203, -21.474) -> (62.3561, -21.474)
  line L15 (61.6016, -21.3273) -> (60.2851, -2.5) projected
  line L16 (62.3561, -21.474) -> (61.6016, -21.3273)
  line L17 (61.6016, -21.3273) -> (60.2851, -2.5)
  line L18 (18.5, -2.5) -> (8, -13) projected
  line L19 (60.2851, -2.5) -> (18.5, -2.5)
  line L20 (18.5, -2.5) -> (8, -13)
  line L21 (-3.5, -13) -> (-63.5, -13) projected
  line L22 (8, -13) -> (-3.5, -13)
  line L23 (-3.5, -13) -> (-3.5, -10)
  line L24 (5, -10) -> (-72, -10) projected
  line L25 (-3.5, -10) -> (5, -10)
  line L26 (5, -5) -> (-72, -5) projected
  line L27 (5, -10) -> (5, -5)
  line L28 (5, -5) -> (0, -5)
  line L29 (0, -5) -> (-67, -5) projected
  line L30 (0, 0) -> (-67, 0) projected
  line L31 (0, -5) -> (0, 0)
  line L32 (62.7851, 0) -> (62.89, -1.5) projected
  line L33 (0, 0) -> (62.7851, 0)
  line L34 (62.89, -1.5) -> (64.0058, -17.4574) projected
  line L35 (62.7851, 0) -> (64.0058, -17.4574)
  line L36 (104.499, -25.8378) -> (104.5905, -25.3462) projected
  line L37 (64.0058, -17.4574) -> (104.5905, -25.3462)
  line L38 (104.5905, -25.3462) -> (104.4405, -26.1524)
  line L39 (-144.5189, -40.3035) -> (-143.0168, -40.2247) projected
  line L40 (-143.5851, -37.7629) -> (-143.6454, -36.8932) projected
  line L41 (-143.0168, -40.2247) -> (-143.5851, -37.7629)
  line L42 (-143.5851, -37.7629) -> (-146.0292, -2.5)
  line L43 (-144.6236, -22.7796) -> (-143.6454, -36.8932) projected
  line L44 (-144.2292, 0) -> (-144.2292, -2.5) projected
  line L45 (-146.0292, -2.5) -> (-144.2292, -2.5)
  line L46 (-144.2292, -2.5) -> (-144.2292, 0)
  line L47 (-146.5812, -37.8675) -> (-149.2292, 0) projected
  line L48 (-144.2292, 0) -> (-149.2292, 0)
  line L49 (-145.0812, -37.8675) -> (-146.5812, -37.8675) projected
  line L50 (-149.2292, 0) -> (-146.5812, -37.8675)
  line L51 (-146.5812, -37.8675) -> (-145.0812, -37.8675)
  line L52 (-143.0168, -40.2247) -> (-144.5189, -40.3035) projected
  line L53 (-143.0168, -40.2247) -> (-144.5189, -40.3035)
  line L54 (-145.0812, -37.8675) -> (-144.5189, -40.3035) projected
  line L55 (-145.0812, -37.8675) -> (-144.5189, -40.3035)
  line L56 (-144.5189, -40.3035) -> (-143.0168, -40.2247)
  line L57 (-87.4292, 0) -> (-87.4292, -2.5) projected
  line L58 (-67, 0) -> (-67, -5) projected
  line L59 (-87.4292, 0) -> (-67, 0)
  line L60 (-67, 0) -> (-67, -5)
  line L61 (-67, -5) -> (-72, -5) projected
  line L62 (-67, -5) -> (-72, -5)
  line L63 (-72, -5) -> (-72, -10) projected
  line L64 (-72, -5) -> (-72, -10)
  line L65 (-63.5, -10) -> (-63.5, -13) projected
  line L66 (-72, -10) -> (-63.5, -10)
  line L67 (-63.5, -10) -> (-63.5, -13)
  line L68 (8, -13) -> (-75, -13) projected
  line L69 (-63.5, -13) -> (-75, -13)
  line L70 (-75, -13) -> (-85.5, -2.5) projected
  line L71 (-75, -13) -> (-85.5, -2.5)
  line L72 (-85.5, -2.5) -> (-87.4292, -2.5)
  line L73 (-87.4292, -2.5) -> (-87.4292, 0)
  point P0 (62.7851, -2.5)
  constraints: 84 end point, 19 collinear, 10 perpendicular, 4 parallel, 3 point on line, 2 horizontal, 1 vertical
extrude "Extrusion31" add sketch "Sketch42" along normal blind 7.5 contours L2 L1 L4 L3 L6 L7 L9 L12 L11 L16 L15 L19 L18 L22 L23 L24 L27 L26 L31 L33 L32 L34 L0 | L58 L26 L63 L24 L65 L68 L70 L72 L57 L59 | L54 L49 L47 L48 L44 L45 L42 L40 L41 L39
sketch "Sketch43" plane through (0, 2.5, 0) normal (0, 1, 0) x (1, 0, 0)
  arc A0 (-70, 62.7851) -> (-70, 129.7851) centre (-70, 96.2851) ccw projected
  line L0 (-70, 129.7851) -> (-70, 96.2851)
  line L1 (-70, 96.2851) -> (-77.5, 96.2851)
  line L2 (-70, 129.7851) -> (-77.5, 129.7851) projected
  line L3 (-77.5, 96.2851) -> (-77.5, 129.7851)
  circle A1 centre (-77.5, 96.2851) radius 33.5
  circle A2 centre (-70, 96.2851) radius 33.5
  line L4 (-77.5, 66.2851) -> (-77.5, 54.7851) projected
  line L5 (-77.5, 62.7851) -> (-70, 62.7851)
  point P0 (0, 0)
  point P1 (-73.75, 62.9956)
  dimension "d161" = 7.5
  constraints: 8 end point, 2 centre point, 2 coincident, 2 point on circle, 1 concentric, 1 perpendicular, 1 point on line, 1 tangent, 1 vertical
  measures "d161" distance of L0.end L1.end
extrude "Extrusion32" add sketch "Sketch43" against normal blind 5 contours A2 A1 L0 A0 | L5 A1 A2 | A2 A1 L2 | L0 A1 A2
sketch "Sketch44" plane through (-70, -7.5, -96.2851) normal (0, 1, 0) x (1, 0, 0)
  arc A0 (-7.5, -33.5) -> (-7.5, 33.5) centre (-7.5, 0) ccw projected
  line L0 (26, 0) -> (0, 0)
  line L1 (0, 30) -> (-7.5, 30) projected
  line L2 (0, 0) -> (0, 30)
  line L3 (0, 30) -> (0, 0)
  arc A1 (0, -38.5) -> (0, 38.5) centre (0, 0) ccw projected
  line L4 (-7.5, 30) -> (-7.5, 38.5) projected
  line L5 (-7.5, 30) -> (-7.5, 0)
  circle A2 centre (-7.5, 0) radius 38.5
  circle A3 centre (-7.5, 0) radius 30
  line L6 (-7.5, 38.5) -> (0, 38.5)
  line L7 (-7.5, -38.5) -> (-7.5, -30) projected
  line L8 (0, -38.5) -> (-7.5, -38.5) projected
  line L9 (-7.5, -38.5) -> (0, -38.5)
  circle A4 centre (0, 0) radius 38.5
  point P0 (70, -96.2851)
  constraints: 12 end point, 4 point on circle, 3 centre point, 3 coincident, 2 perpendicular, 1 collinear, 1 horizontal, 1 parallel, 1 tangent, 1 vertical
extrude "Extrusion33" add sketch "Sketch44" along normal blind 5 contours A2 A4 L8 | A2 A4 A1 | L6 A4 A2
sketch "Sketch45" plane through (-70, -7.5, -96.2851) normal (0, 1, 0) x (1, 0, 0)
  arc A0 (0, -30) -> (0, 30) centre (0, 0) ccw projected
  line L0 (0, 0) -> (0, 30)
  line L1 (0, 30) -> (0, 0)
  line L2 (0, 0) -> (-7.5, 0)
  line L3 (-7.5, 30) -> (-7.5, 38.5) projected
  line L4 (-7.5, 0) -> (-7.5, 38.5)
  line L5 (-7.5, 38.5) -> (-7.5, 0)
  line L6 (0, 30) -> (-7.5, 30) projected
  circle A1 centre (-7.5, 0) radius 30
  circle A2 centre (0, 0) radius 30
  line L7 (0, 30) -> (-7.5, 30) projected
  line L8 (-7.5, 30) -> (0, 30)
  line L9 (0, -30) -> (-7.5, -30) projected
  line L10 (0, 30) -> (0, -30)
  line L11 (0, -30) -> (-7.5, -30)
  point P0 (70, -96.2851)
  constraints: 16 end point, 3 collinear, 3 horizontal, 3 perpendicular, 2 coincident, 2 tangent, 1 centre point, 1 point on circle, 1 vertical, 1 vertical alignment, 2 other
extrude "Extrusion34" add sketch "Sketch45" against normal blind 3 contours L10 A1 L0 A0 | L9 A1 A2 | A2 A1 L10 | A2 A1 L6 | L0 A1 A2
sketch "Sketch47" plane through (-70, -10.5, -96.2851) normal (0, -1, 0) x (1, 0, 0)
  arc A0 (-7.5, -30) -> (-7.5, 30) centre (-7.5, 0) ccw projected
  line L0 (-7.5, -30) -> (-7.5, -38.5)
  line L1 (-7.5, -41.5) -> (-7.5, -30) projected
  line L2 (-7.5, 38.5) -> (-7.5, 30) projected
  line L3 (-7.5, 38.5) -> (-7.5, 30)
  circle A1 centre (-7.5, 0) radius 30
  circle A2 centre (-7.5, 0) radius 38.5
  circle A3 centre (-7.5, 0) radius 41.5
  point P0 (70, 96.2851)
  point P1 (-7.5, -38.5)
  dimension "d168" = 8.5
  constraints: 4 end point, 3 coincident, 2 vertical alignment, 1 point on line, 1 vertical, 7 other
  measures "d168" distance of L0.start L0.end
extrude "Extrusion35" cut sketch "Sketch47" against normal blind 3 contours A0 L2 A2 L0 | A3
sketch "Sketch48" plane through (-70, -10.5, -96.2851) normal (0, -1, 0) x (1, 0, 0)
  arc A0 (-7.5, -33.5) -> (-7.5, 33.5) centre (-7.5, 0) ccw projected
  line L0 (-7.5, -52) -> (-7.5, -41.5) projected
  circle A1 centre (-7.5, 0) radius 41.5
  arc A2 (-7.5, -41.5) -> (-7.5, 41.5) centre (-7.5, 0) ccw projected
  line L1 (34, 0) -> (38, 0)
  circle A3 centre (-7.5, 0) radius 45.5
  point P0 (70, 96.2851)
  dimension "d171" = 4
  constraints: 2 coincident, 2 end point, 2 point on circle, 1 centre point, 1 horizontal, 1 horizontal alignment, 2 other
  measures "d171" distance of L1.start L1.end
extrude "Extrusion36" cut sketch "Sketch48" against normal blind 8 contours A3 L1 A1 L0 | L0 A1 L1 A3
sketch "Sketch49" plane through (0, 2.5, 0) normal (0, 1, 0) x (1, 0, 0)
  line L0 (-22.5, 150.2143) -> (-77.5, 150.2143) projected
  line L1 (-22.5, 150.2143) -> (-22.5, 144.2143)
  line L2 (-22.5, 144.2143) -> (-27.5, 144.2143)
  line L3 (-27.5, 144.2143) -> (-27.5, 150.2143)
  point P0 (0, 0)
  dimension "d174" = 6
  dimension "d175" = 5
  constraints: 6 end point, 2 perpendicular, 1 point on line, 1 vertical
  measures "d174" distance of L0.start L1.end
  measures "d175" distance of L1.end L2.end
extrude "Extrusion37" cut sketch "Sketch49" against normal blind 2
mirror "Mirror4" about plane through (-77.5, -11.8458, -12.2398) normal (-1, 0, 0)
sketch "Sketch51" plane through (-70, -10.5, -96.2851) normal (0, -1, 0) x (1, 0, 0)
  line L0 (48, -41.5) -> (11.1548, -41.5) projected
  line L1 (48, -41.5) -> (24, -41.5)
  line L2 (24, -41.5) -> (24, -52)
  line L3 (-63, -52) -> (48, -52) projected
  line L4 (24, -52) -> (22, -52)
  line L5 (22, -52) -> (22, -41.5)
  line L6 (22, -41.5) -> (24, -41.5)
  circle A0 centre (-7.5, 0) radius 33.5 projected
  line L7 (-7.5, -33.5) -> (-7.5, 33.5)
  line L8 (-7.5, 0) -> (26, 0)
  line L9 (-63, -41.5) -> (-26.1548, -41.5)
  line L10 (-39, -41.5) -> (-39, -52)
  line L11 (48, -52) -> (-63, -52)
  line L12 (-37, -52) -> (-37, -41.5)
  line L13 (24, 41.5) -> (24, 52)
  line L14 (-63, 52) -> (48, 52)
  line L15 (22, 52) -> (22, 41.5)
  line L16 (22, 41.5) -> (24, 41.5)
  line L17 (-37, 52) -> (-37, 41.5)
  line L18 (-39, 41.5) -> (-39, 52)
  line L19 (-63, 41.5) -> (-26.1548, 41.5)
  point P0 (70, 96.2851)
  point P1 (-37, 41.5)
  point P2 (-37, 52)
  point P3 (-37, -41.5)
  point P4 (-37, -52)
  dimension "d181" = 24
  dimension "d182" = 2
  constraints: 36 end point, 20 symmetric about line, 10 point on line, 4 perpendicular, 3 point on circle, 1 vertical
  measures "d181" distance of L0.start L1.end
  measures "d182" distance of L2.end L4.end
extrude "Extrusion38" add sketch "Sketch51" along normal blind 20 and the other way blind 12 contours L2 L3 L5 L0 | L10 L9 L12 L3 | L16 L15 L14 L13 | L14 L17 L19 L18
sketch "Sketch52" plane through (0, -26.4938, -209.9869) normal (0, -0.0697565, -0.9975641) x (-1, 0, 0)
  line L0 (2.5, 29.0646) -> (2.5, 5.9999) projected
  line L1 (152.5, 29.0646) -> (152.5, 5.9999) projected
  line L2 (2.5, 29.0646) -> (152.5, 29.0646)
  line L3 (152.5, 29.0646) -> (77.5, 29.0646)
  line L4 (2.5, 29.0646) -> (152.5, 29.0646) projected
  line L5 (77.5, 29.0646) -> (77.5, -9)
  line L6 (132.8, -9) -> (22.2, -9) projected
  line L7 (77.5, 29.0646) -> (77.5, 24.0646)
  line L8 (77.5, 24.0646) -> (89.5, 24.0646)
  line L9 (89.5, 24.0646) -> (89.5, 14.0646)
  line L10 (89.5, 14.0646) -> (99.5, 14.0646)
  line L11 (99.5, 14.0646) -> (99.5, 24.0646)
  line L12 (99.5, 24.0646) -> (89.5, 24.0646)
  line L13 (77.5, 24.0646) -> (65.5, 24.0646)
  line L14 (65.5, 24.0646) -> (65.5, 14.0646)
  line L15 (65.5, 14.0646) -> (55.5, 14.0646)
  line L16 (55.5, 14.0646) -> (55.5, 24.0646)
  line L17 (55.5, 24.0646) -> (65.5, 24.0646)
  point P0 (0, 11.7814)
  dimension "d187" = 5
  dimension "d188" = 12
  dimension "d189" = 10
  dimension "d190" = 10
  constraints: 28 end point, 4 symmetric about line, 3 perpendicular, 3 point on line, 2 horizontal, 2 midpoint, 1 collinear
  measures "d187" distance of L3.end L7.end
  measures "d188" distance of L7.end L8.end
  measures "d189" distance of L8.end L9.end
  measures "d190" distance of L9.end L10.end
extrude "Extrusion39" cut sketch "Sketch52" against normal blind 20
body "Solid1"
